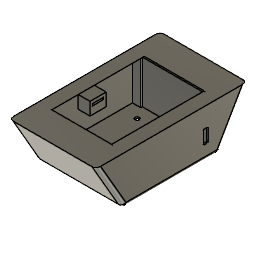
261L Project Housing (Autodesk Fusion 360 design; units mm, degrees)
Autodesk Fusion 360 part; units mm, degrees
sketch "Servo Arm" plane through (0, 0, 0) normal (0, 0, 1) x (1, 0, 0)
  line L0 (0, 0) -> (0, -20.25)
  line L1 (0, 0) -> (-3.75, 0)
  line L2 (-3.75, 0) -> (-3.75, -46.1)
  line L3 (-3.75, 0) -> (-6.6, 0)
  line L4 (-6.6, 0) -> (-6.6, 3.1)
  line L5 (-6.6, 3.1) -> (-3.75, 3.1)
  line L6 (-3.75, 3.1) -> (-3.75, 0)
  line L7 (-3.75, -46.1) -> (-6.6, -46.1)
  line L8 (-6.6, -46.1) -> (-6.6, -49.2)
  line L9 (-6.6, -49.2) -> (-3.75, -49.2)
  line L10 (-3.75, -49.2) -> (-3.75, -46.1)
  line L11 (-3.75, 3.1) -> (0, 3.1)
  line L12 (0, 3.1) -> (0, 0)
  line L13 (0, -20.25) -> (15, -20.25)
  line L14 (0, -20.25) -> (0, -49.2)
  line L15 (0, -49.2) -> (-3.75, -49.2)
  line L16 (0, 0) -> (3, 0)
  line L17 (0, -20.25) -> (3, -20.25)
  line L18 (3, 0) -> (3, -20.25)
  line L19 (15, -20.25) -> (15, -23.25)
  line L20 (15, -23.25) -> (0, -23.25)
  line L21 (0, 0) -> (15, 0)
  line L22 (15, 0) -> (15, 3.15)
  line L23 (15, 3.15) -> (0, 3.1)
  dimension "d1" = 20.25
  dimension "d2" = 46.1
  dimension "d3" = 3.75
  dimension "d4" = 3.1
  dimension "d5" = 2.85
  dimension "d6" = 3.1
  dimension "d7" = 2.85
  dimension "d8" = 15
  dimension "d9" = 3
  dimension "d10" = 3
  dimension "d11" = 15
  dimension "d12" = 3.15
  constraint coincident L0.start L1.start
  constraint vertical L0
  constraint perpendicular L0 L1
  constraint perpendicular L1 L2
  constraint horizontal L3
  constraint vertical L4
  constraint horizontal L5
  constraint vertical L6
  constraint horizontal L7
  constraint vertical L8
  constraint horizontal L9
  constraint vertical L10
  constraint perpendicular L0 L11
  constraint perpendicular L1 L12
  constraint perpendicular L0 L13
  constraint perpendicular L13 L14
  constraint perpendicular L10 L15
  constraint perpendicular L0 L16
  constraint coincident L13 L17.end
  constraint perpendicular L13 L19
  constraint coincident L14 L20.end
  constraint perpendicular L14 L20
  constraint perpendicular L12 L21
  constraint perpendicular L21 L22
  measures "d1" distance of L0.start L0.end
  measures "d2" distance of L1.end L2.end
  measures "d3" distance of L0.start L1.end
  measures "d4" distance of L1.end L5.end
  measures "d5" distance of L1.end L3.end
  measures "d6" distance of L2.end L9.end
  measures "d7" distance of L8.end L9.end
  measures "d8" distance of L0.end L13.end
  measures "d9" distance of L0.start L16.end
  measures "d10" distance of L13.end L19.end
  measures "d11" distance of L0.start L21.end
  measures "d12" distance of L21.end L22.end
extrude "Extrude1" add sketch "Servo Arm" along normal blind 4.45 contours L0 L13 L16 L17 L18 L21 | L3 L4 L5 L6 | L7 L8 L9 L10 makes body 1 at (-6.6, 1.0333, 1.4833) makes body 2 at (3, -6.75, 2.9667) makes body 3 at (-3.75, -47.1333, 2.9667)
extrude "Extrude2" add sketch "Servo Arm" against normal blind 5 bodies 1 2 3
sketch "Housing Bottom Profile" plane through (0, 0, 0) normal (0, 0, 1) x (1, 0, 0)
  line L0 (0, 0) -> (-107, 0)
  line L1 (-107, 0) -> (-107, 116)
  line L2 (-107, 116) -> (0, 116)
  line L3 (0, 116) -> (0, 0)
  line L4 (0, 0) -> (-2, 0)
  line L5 (-2, 0) -> (-2, 116)
  line L6 (0, 116) -> (0, 118)
  line L7 (0, 118) -> (-107, 118)
  line L8 (-107, 118) -> (-109, 118)
  line L9 (-109, 118) -> (-109, 0)
  line L10 (-109, 0) -> (-109, -2)
  line L11 (-109, -2) -> (0, -2)
  line L12 (0, -2) -> (0, 0)
  line L13 (-2, 116) -> (-107, 116)
  line L14 (-54.5, 116) -> (-54.5, 2)
  line L15 (-54.5, 116) -> (-19.5, 116)
  line L16 (-54.5, 116) -> (-89.5, 116)
  line L17 (-19.5, 116) -> (-19.5, 0)
  line L18 (-89.5, 116) -> (-89.5, 0)
  line L19 (-54.5, 2) -> (-19.5, 2)
  line L20 (-54.5, 2) -> (-89.5, 2)
  line L21 (-54.5, 116) -> (-50, 116)
  line L22 (-54.5, 116) -> (-59, 116)
  line L23 (-50, 116) -> (-50, 2)
  dimension "d17" = 107
  dimension "d18" = 116
  dimension "d25" = 2
  dimension "d26" = 2
  dimension "d27" = 2
  dimension "d28" = 2
  dimension "d56" = 114
  dimension "d57" = 35
  dimension "d58" = 35
  dimension "d59" = 4.5
  dimension "d60" = 4.5
  constraint horizontal L0
  constraint vertical L1
  constraint horizontal L2
  constraint vertical L3
  constraint coincident L0.start L3.end
  constraint perpendicular L3 L4
  constraint coincident L2 L5.end
  constraint perpendicular L2 L5
  constraint vertical L6
  constraint perpendicular L1 L7
  constraint perpendicular L3 L8
  constraint perpendicular L0 L9
  constraint perpendicular L0 L10
  constraint perpendicular L3 L11
  constraint perpendicular L4 L12
  constraint midpoint L13 L14.start
  constraint perpendicular L2 L14
  constraint perpendicular L14 L15
  constraint perpendicular L14 L16
  constraint coincident L0 L17.end
  constraint perpendicular L0 L17
  constraint coincident L0 L18.end
  constraint perpendicular L0 L18
  constraint coincident L17 L19.end
  constraint perpendicular L17 L19
  constraint coincident L18 L20.end
  constraint perpendicular L18 L20
  constraint perpendicular L14 L21
  constraint perpendicular L14 L22
  constraint coincident L19 L23.end
  constraint perpendicular L19 L23
  measures "d17" distance of L0.start L0.end
  measures "d18" distance of L0.start L2.end
  measures "d25" distance of L0.start L4.end
  measures "d26" distance of L2.end L6.end
  measures "d27" distance of L7.end L8.end
  measures "d28" distance of L9.end L10.end
  measures "d56" distance of L14.start L14.end
  measures "d57" distance of L14.start L15.end
  measures "d58" distance of L14.start L16.end
  measures "d59" distance of L14.start L21.end
  measures "d60" distance of L14.start L22.end
sketch "Housing Side Profile" plane through (0, 0, 0) normal (1, 0, 0) x (0, 1, 0)
  line L0 (0, 0) -> (116, 0)
  line L1 (116, 0) -> (116, 58)
  line L2 (116, 58) -> (0, 58)
  line L3 (0, 58) -> (0, 0)
  line L4 (116, 0) -> (116, 2)
  line L5 (116, 2) -> (0, 2)
  line L6 (0, 0) -> (-2, 0)
  line L7 (-2, 0) -> (-2, 58)
  line L8 (-2, 58) -> (0, 58)
  line L9 (-2, 58) -> (-2, 60)
  line L10 (118, 60) -> (118, 0)
  line L11 (118, 0) -> (116, 0)
  line L12 (-2, 0) -> (-36.641, 60)
  line L13 (-36.641, 60) -> (-2, 60)
  line L14 (118, 0) -> (152.641, 60)
  line L15 (152.641, 60) -> (118, 60)
  line L16 (-2, 60) -> (118, 60)
  line L17 (116, 58) -> (118, 58)
  dimension "d19" = 116
  dimension "d20" = 58
  dimension "d21" = 2
  dimension "d22" = 2
  dimension "d23" = 2
  dimension "d39" = 120
  dimension "d47" = 120
  dimension "d48" = 2
  constraint horizontal L0
  constraint vertical L1
  constraint horizontal L2
  constraint vertical L3
  constraint coincident L0.start L3.end
  constraint perpendicular L0 L4
  constraint coincident L3 L5.end
  constraint perpendicular L3 L5
  constraint perpendicular L3 L6
  constraint perpendicular L2 L7
  constraint perpendicular L3 L8
  constraint perpendicular L8 L9
  constraint perpendicular L0 L10
  constraint perpendicular L1 L11
  constraint perpendicular L9 L13
  constraint perpendicular L10 L15
  constraint perpendicular L10 L16
  constraint coincident L10 L17.end
  constraint perpendicular L10 L17
  measures "d19" distance of L1.end L2.end
  measures "d20" distance of L0.start L2.end
  measures "d21" distance of L0.end L4.end
  measures "d22" distance of L0.start L6.end
  measures "d23" distance of L7.end L9.end
  measures "d39" angle of L6 L12
  measures "d47" angle of L11 L14
  measures "d48" distance of L1.end L17.end
extrude "Extrude3" add sketch "Housing Bottom Profile" along normal blind 60 separate body contours L0 L1 L2 L4 L6 L7 L8 L9 L10 L11 L12 L13 L15 L16 L21 L22 | L0 L2 L3 L4 L5 makes body 4
extrude "Extrude4" add sketch "Housing Bottom Profile" along normal blind 2 contours L0 L2 L5 L13 L17 | L0 L17 L18 L19 L20 | L0 L1 L2 L13 L18 | L2 L13 L15 L17 L19 L23 | L2 L13 L14 L16 L18 L20 L22 | L2 L13 L14 L15 L19 L21 L23 bodies 4
sketch "Command Strip Bars" plane through (0, 116, 0) normal (0, -1, 0) x (1, 0, 0)
  line L0 (-107, 2) -> (-2, 2)
  line L1 (-2, 2) -> (-2, 60)
  line L2 (-2, 60) -> (-107, 60)
  line L3 (-107, 60) -> (-107, 2)
  line L4 (-2, 60) -> (-2, 52)
  line L5 (-107, 60) -> (-107, 52)
  line L6 (-107, 60) -> (-92, 60)
  line L7 (-107, 52) -> (-92, 60)
  line L8 (-2, 60) -> (-17, 60)
  line L9 (-17, 60) -> (-2, 52)
  line L10 (-2, 60) -> (-2, 58)
  line L11 (-2, 58) -> (-107, 58)
  line L12 (-54.5, 58) -> (-54.5, 2)
  line L13 (-54.5, 58) -> (-12.5, 58)
  line L14 (-54.5, 58) -> (-96.5, 58)
  line L15 (-12.5, 58) -> (-12.5, 2)
  line L16 (-96.5, 58) -> (-96.5, 2)
  line L17 (-96.5, 2) -> (-12.5, 2)
  dimension "d33" = 8
  dimension "d34" = 8
  dimension "d35" = 15
  dimension "d36" = 15
  dimension "d45" = 2
  dimension "d46" = 90
  dimension "d49" = 56
  dimension "d50" = 42
  dimension "d51" = 42
  constraint coincident L1.end L2.start
  constraint perpendicular L2 L4
  constraint coincident L2.end L3.start
  constraint perpendicular L2 L5
  constraint perpendicular L3 L6
  constraint perpendicular L1 L8
  constraint perpendicular L2 L10
  constraint coincident L5 L11.end
  constraint midpoint L11 L12.start
  constraint perpendicular L11 L12
  constraint perpendicular L12 L13
  constraint perpendicular L12 L14
  constraint coincident L0 L15.end
  constraint perpendicular L0 L15
  constraint coincident L0 L16.end
  constraint perpendicular L0 L16
  measures "d33" distance of L1.end L4.end
  measures "d34" distance of L2.end L5.end
  measures "d35" distance of L2.end L6.end
  measures "d36" distance of L1.end L8.end
  measures "d45" distance of L1.end L10.end
  measures "d46" angle of L5 L11
  measures "d49" distance of L12.start L12.end
  measures "d50" distance of L12.start L13.end
  measures "d51" distance of L12.start L14.end
extrude "Extrude5" add sketch "Command Strip Bars" along normal blind 116 contours L3 L5 L7 L11 L16 | L7 L11 L14 L16 | L2 L3 L5 L6 L7 L11 L14 | L1 L4 L9 L11 L15 | L9 L11 L13 L15 | L1 L2 L4 L8 L9 L10 L11 L13 bodies 4
extrude "Extrude6" add sketch "Housing Side Profile" against normal blind 109 contours L7 L9 L12 L13 | L10 L14 L15 bodies 4
fillet "Fillet1" radius 5 8 edges at (0, -19.3205, 30) (-54.5, -2, 0) (-109, -19.3205, 30) (0, 58, 0) (-109, 58, 0) (-109, 135.3205, 30) (-54.5, 118, 0) (0, 135.3205, 30) on bodies 4
extrude "Extrude7" cut sketch "Command Strip Bars" along normal blind 116 and the other way blind 2 contours L0 L7 L11 L12 L14 L16 L17 | L0 L9 L11 L12 L13 L15 L17 | L7 L11 L14 L16 | L9 L11 L13 L15 bodies 4
sketch "Servo Attachment Point" plane through (-107, 0, 0) normal (1, 0, 0) x (0, 1, 0)
  line L0 (116, 52) -> (0, 52)
  line L1 (0, 52) -> (0, 2)
  line L2 (0, 2) -> (116, 2)
  line L3 (116, 2) -> (116, 52)
  line L4 (116, 2) -> (0, 2)
  line L5 (58, 2) -> (58, 52)
  line L6 (58, 52) -> (48, 52)
  line L7 (58, 52) -> (68, 52)
  line L8 (58, 52) -> (64.1, 52)
  line L9 (58, 52) -> (51.9, 52)
  line L10 (58, 60) -> (58, 54.9)
  line L11 (58, 54.9) -> (58, 41.24)
  line L12 (58, 41.24) -> (58, 45.24)
  line L13 (58, 41.24) -> (58, 38.74)
  line L14 (58, 38.74) -> (58, 29.24)
  line L15 (58, 45.24) -> (64.1, 45.24)
  line L16 (58, 45.24) -> (51.9, 45.24)
  line L17 (51.9, 45.24) -> (51.9, 41.24)
  line L18 (51.9, 41.24) -> (64.1, 41.24)
  line L19 (64.1, 41.24) -> (64.1, 45.24)
  line L20 (64.1, 41.24) -> (64.1, 38.74)
  line L21 (64.1, 38.74) -> (51.9, 38.74)
  line L22 (51.9, 38.74) -> (51.9, 41.24)
  line L23 (51.9, 38.74) -> (51.9, 29.24)
  line L24 (51.9, 29.24) -> (64.1, 29.24)
  line L25 (64.1, 29.24) -> (64.1, 38.74)
  line L26 (64.1, 45.24) -> (68.1, 45.24)
  line L27 (51.9, 45.24) -> (47.9, 45.24)
  line L28 (64.1, 29.24) -> (68.1, 29.24)
  line L29 (68.1, 29.24) -> (68.1, 45.24)
  line L30 (51.9, 29.24) -> (47.9, 29.24)
  line L31 (47.9, 29.24) -> (47.9, 45.24)
  line L32 (51.9, 41.24) -> (50.9, 41.24)
  line L33 (51.9, 38.74) -> (50.9, 38.74)
  line L34 (50.9, 38.74) -> (50.9, 41.24)
  line L35 (64.1, 38.74) -> (65.1, 38.74)
  line L36 (64.1, 41.24) -> (65.1, 41.24)
  line L37 (65.1, 41.24) -> (65.1, 38.74)
  dimension "d61" = 10
  dimension "d62" = 10
  dimension "d63" = 6.1
  dimension "d64" = 6.1
  dimension "d65" = 5.1
  dimension "d66" = 13.66
  dimension "d67" = 4
  dimension "d68" = 2.5
  dimension "d69" = 9.5
  dimension "d77" = 4
  dimension "d78" = 4
  dimension "d79" = 4
  dimension "d80" = 4
  dimension "d81" = 1
  dimension "d82" = 1
  dimension "d83" = 1
  dimension "d84" = 1
  constraint coincident L2.end L3.start
  constraint coincident L1.end L2.start
  constraint midpoint L2 L5.start
  constraint midpoint L0 L5.end
  constraint perpendicular L5 L6
  constraint perpendicular L5 L7
  constraint perpendicular L5 L8
  constraint perpendicular L5 L9
  constraint vertical L10
  constraint parallel L5 L11
  constraint parallel L11 L12
  constraint parallel L5 L13
  constraint parallel L5 L14
  constraint perpendicular L12 L15
  constraint perpendicular L12 L16
  constraint perpendicular L16 L17
  constraint perpendicular L11 L18
  constraint perpendicular L18 L19
  constraint perpendicular L18 L20
  constraint perpendicular L17 L21
  constraint perpendicular L18 L22
  constraint perpendicular L21 L23
  constraint perpendicular L20 L24
  constraint perpendicular L21 L25
  constraint perpendicular L19 L26
  constraint perpendicular L17 L27
  constraint perpendicular L25 L28
  constraint perpendicular L23 L30
  constraint perpendicular L17 L32
  constraint perpendicular L22 L33
  constraint perpendicular L25 L35
  constraint perpendicular L19 L36
  measures "d61" distance of L5.end L6.end
  measures "d62" distance of L5.end L7.end
  measures "d63" distance of L5.end L8.end
  measures "d64" distance of L5.end L9.end
  measures "d65" distance of L10.start L10.end
  measures "d66" distance of L10.end L11.end
  measures "d67" distance of L11.end L12.end
  measures "d68" distance of L11.end L13.end
  measures "d69" distance of L13.end L14.end
  measures "d77" distance of L15.end L26.end
  measures "d78" distance of L16.end L27.end
  measures "d79" distance of L24.end L28.end
  measures "d80" distance of L23.end L30.end
  measures "d81" distance of L17.end L32.end
  measures "d82" distance of L21.end L33.end
  measures "d83" distance of L20.end L35.end
  measures "d84" distance of L18.end L36.end
extrude "Extrude8" add sketch "Servo Attachment Point" along normal blind 9.85 contours L5 L13 L18 L21 L22 | L5 L13 L18 L20 L21 | L20 L35 L36 L37 | L22 L32 L33 L34 bodies 4
extrude "Extrude9" add sketch "Servo Attachment Point" along normal blind 15 contours L5 L14 L21 L23 L24 | L5 L14 L21 L24 L25 | L5 L11 L12 L15 L18 L19 | L5 L11 L12 L16 L17 L18 | L17 L23 L27 L30 L31 L32 L33 L34 | L19 L25 L26 L28 L29 L35 L36 L37 bodies 4
sketch "Sketch6" plane through (0, 0, 2) normal (0, 0, 1) x (-1, 0, 0)
  line L0 (96.5, -116) -> (107, -116)
  line L1 (107, -116) -> (107, 0)
  line L2 (107, 0) -> (2, 0)
  line L3 (2, 0) -> (2, -116)
  line L4 (2, -116) -> (12.5, -116)
  line L5 (12.5, -116) -> (12.5, -118)
  line L6 (12.5, -118) -> (96.5, -118)
  line L7 (96.5, -118) -> (96.5, -116)
  line L8 (107, -116) -> (107, -102)
  line L9 (107, -102) -> (87, -102)
  circle A0 centre (87, -102) radius 2.65
  line L10 (107, -116) -> (2, -116)
  line L11 (54.5, -116) -> (54.5, 0)
  line L12 (54.5, -58) -> (63.1006, -58)
  line L13 (69.5, -28) -> (39.5, -28)
  line L14 (39.5, -28) -> (39.5, -88)
  line L15 (39.5, -88) -> (69.5, -88)
  line L16 (69.5, -88) -> (69.5, -28)
  line L17 (69.5, -28) -> (39.5, -88) construction
  line L18 (39.5, -28) -> (69.5, -88) construction
  point P0 (54.5, -58)
  dimension "d74" = 14
  dimension "d75" = 20
  dimension "d76" = 5.3
  dimension "d105" = 60
  dimension "d106" = 30
  constraint coincident L0.end L1.start
  constraint perpendicular L0 L8
  constraint perpendicular L8 L9
  constraint coincident L9.end A0.centre
  constraint coincident L3.end L4.start
  constraint midpoint L10 L11.start
  constraint midpoint L2 L11.end
  constraint midpoint L11 P0
  constraint perpendicular L11 L12
  constraint horizontal L13
  constraint perpendicular L13 L14
  constraint parallel L13 L15
  constraint parallel L14 L16
  constraint coincident L17 P0
  constraint coincident L18 P0
  constraint coincident P0 L12.start
  measures "d74" distance of L0.end L8.end
  measures "d75" distance of L8.end L9.end
  measures "d76" diameter of A0
  measures "d105" distance of L13.end L14.end
  measures "d106" distance of L13.start L13.end
sketch "Sketch7" plane through (-2, 0, 0) normal (-1, 0, 0) x (0, -1, 0)
  line L0 (0, 52) -> (-116, 52)
  line L1 (-116, 52) -> (-116, 2)
  line L2 (-116, 2) -> (0, 2)
  line L3 (0, 2) -> (0, 52)
  line L4 (-116, 27) -> (-106, 27)
  line L5 (-106, 27) -> (-101, 27)
  line L6 (-101, 27) -> (-104, 27)
  line L7 (-101, 27) -> (-98, 27)
  line L8 (-98, 27) -> (-98, 35.5)
  line L9 (-104, 27) -> (-104, 18.5)
  line L10 (-98, 35.5) -> (-104, 35.5)
  line L11 (-104, 35.5) -> (-104, 18.5)
  line L12 (-104, 18.5) -> (-98, 18.5)
  line L13 (-98, 18.5) -> (-98, 35.5)
  line L14 (-104, 35.5) -> (-104, 34.5)
  line L15 (-104, 34.5) -> (-103, 34.5)
  line L16 (-103, 34.5) -> (-103, 35.5)
  line L17 (-98, 35.5) -> (-99, 35.5)
  line L18 (-99, 35.5) -> (-99, 34.5)
  line L19 (-99, 34.5) -> (-98, 34.5)
  line L20 (-98, 34.5) -> (-98, 35.5)
  line L21 (-98, 18.5) -> (-99, 18.5)
  line L22 (-99, 18.5) -> (-99, 19.5)
  line L23 (-99, 19.5) -> (-98, 19.5)
  line L24 (-98, 19.5) -> (-98, 18.5)
  line L25 (-104, 18.5) -> (-103, 18.5)
  line L26 (-103, 18.5) -> (-103, 19.5)
  line L27 (-103, 19.5) -> (-104, 19.5)
  line L28 (-104, 19.5) -> (-104, 18.5)
  arc A0 (-104, 19.5) -> (-103, 18.5) centre (-103, 19.5) ccw
  arc A1 (-99, 18.5) -> (-98, 19.5) centre (-99, 19.5) ccw
  arc A2 (-98, 34.5) -> (-99, 35.5) centre (-99, 34.5) ccw
  arc A3 (-103, 35.5) -> (-104, 34.5) centre (-103, 34.5) ccw
  dimension "d87" = 10
  dimension "d88" = 5
  dimension "d89" = 3
  dimension "d90" = 3
  dimension "d91" = 8.5
  dimension "d93" = 8.5
  dimension "d94" = 1
  dimension "d95" = 1
  dimension "d96" = 1
  dimension "d97" = 1
  dimension "d98" = 1
  dimension "d99" = 1
  dimension "d100" = 1
  dimension "d101" = 1
  dimension "d102" = 1
  constraint midpoint L1 L4.start
  constraint perpendicular L1 L4
  constraint parallel L4 L5
  constraint parallel L5 L6
  constraint parallel L6 L7
  constraint perpendicular L7 L8
  constraint perpendicular L6 L9
  constraint horizontal L10
  constraint vertical L11
  constraint horizontal L12
  constraint vertical L13
  constraint perpendicular L10 L14
  constraint perpendicular L14 L15
  constraint perpendicular L10 L16
  constraint horizontal L17
  constraint vertical L18
  constraint horizontal L19
  constraint vertical L20
  constraint horizontal L21
  constraint vertical L22
  constraint horizontal L23
  constraint vertical L24
  constraint horizontal L25
  constraint vertical L26
  constraint horizontal L27
  constraint vertical L28
  measures "d87" distance of L4.start L4.end
  measures "d88" distance of L4.end L5.end
  measures "d89" distance of L5.end L6.end
  measures "d90" distance of L5.end L7.end
  measures "d91" distance of L7.end L8.end
  measures "d93" distance of L6.end L9.end
  measures "d94" distance of L10.end L14.end
  measures "d95" distance of L14.end L15.end
  measures "d96" distance of L15.end L16.end
  measures "d97" distance of L8.end L19.end
  measures "d98" distance of L18.end L19.end
  measures "d99" distance of L12.end L23.end
  measures "d100" distance of L22.end L23.end
  measures "d101" distance of L9.end L27.end
  measures "d102" distance of L26.end L27.end
extrude "Extrude10" cut sketch "Sketch6" against normal blind 40 contours A0 bodies 4
extrude "Extrude11" cut sketch "Sketch7" against normal blind 35 contours L5 L6 L7 L8 L10 L11 L13 L15 L16 L18 L19 | L5 L6 L7 L9 L11 L12 L13 L22 L23 L26 L27 | L26 L27 A0 | L15 L16 A3 | L18 L19 A2 | L22 L23 A1 bodies 4
extrude "Extrude12" cut sketch "Sketch6" against normal blind 70 contours L11 L13 L14 L15 | L11 L13 L15 L16 bodies 4
move_body "Move1" [suppressed]
hidden bodies 1
named bodies: "Servo Arm", "Housing"
